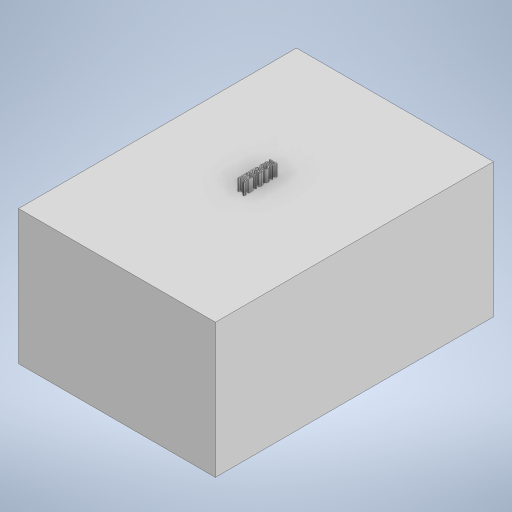
# Autodesk Inventor part: jetson
Saved by Autodesk Inventor 2023 (Build 270158000, 158)
## iProperties
Created: 2022-11-21
Part Number: jetson
Material: Genérico
Document SubType Name: Modeling
Designer: inigo
Density: 1 g/cm^3
Appearance: Valor por defecto
Author: inigo
Autodesk Inventor part; units mm, degrees
ref_plane "YZ Plane" through (0, 0, 0) normal (1, 0, 0) x (0, 1, 0)
ref_plane "XZ Plane" through (0, 0, 0) normal (0, 1, 0) x (-1, 0, 0)
ref_plane "XY Plane" through (0, 0, 0) normal (0, 0, 1) x (1, 0, 0)
sketch "Boceto1" plane through (0, 0, 0) normal (0, 1, 0) x (-1, 0, 0)
  line L0 (42.5, 60) -> (-42.5, 60)
  line L1 (-42.5, 60) -> (-42.5, -60)
  line L2 (-42.5, -60) -> (42.5, -60)
  line L3 (42.5, -60) -> (42.5, 60)
  line L4 (42.5, 60) -> (-42.5, -60) construction
  line L5 (-42.5, 60) -> (42.5, -60) construction
  point P0 (0, 0)
  dimension "d0" = 85
  dimension "d1" = 120
  constraints: 12 end point, 2 midpoint, 2 parallel, 1 horizontal, 1 perpendicular
  measures "d0" distance of L2.end L1.end
  measures "d1" distance of L1.end L0.end
extrude "Extrusión1" add sketch "Boceto1" along normal blind 58
sketch "Boceto2" plane through (0, 58, 0) normal (0, 1, 0) x (1, 0, 0)
  line L0 (-1.6968, -6.642) -> (-1.6968, 31.3478) construction
  line L1 (-1.6968, 31.3478) -> (74.717, 31.3478) construction
  line L2 (74.717, 31.3478) -> (74.717, -6.642) construction
  line L3 (74.717, -6.642) -> (-1.6968, -6.642) construction
  spline S0 degree 2 poles (0.6226, -5.1847) (1.0227, -5.1847) (1.4574, -5.6738) (1.4574, -6.0862) knots 0 0 0 1 2 2 2
  spline S1 degree 2 poles (1.4574, -6.0862) (1.4574, -6.185) (1.4229, -6.5136) (1.3982, -6.6247) knots 0 0 0 1 2 2 2
  line L4 (1.3982, -6.6247) -> (1.0079, -6.6247)
  line L5 (1.0079, -6.6247) -> (1.0079, -6.6025)
  spline S2 degree 2 poles (1.0079, -6.6025) (1.0375, -6.5185) (1.1067, -6.269) (1.1067, -6.1406) knots 0 0 0 1 2 2 2
  spline S3 degree 2 poles (1.1067, -6.1406) (1.1067, -5.9529) (1.0202, -5.7281) (0.9412, -5.6762) knots 0 0 0 1 2 2 2
  spline S4 degree 2 poles (0.9412, -5.6762) (0.8597, -5.6194) (0.6226, -5.5898) (0.467, -5.5898) knots 0 0 0 1 2 2 2
  line L6 (0.467, -5.5898) -> (-1.309, -5.5898)
  line L7 (-1.309, -5.5898) -> (-1.309, -6.2344)
  line L8 (-1.309, -6.2344) -> (-1.6326, -6.2344)
  line L9 (-1.6326, -6.2344) -> (-1.6326, -5.1847)
  line L10 (-1.6326, -5.1847) -> (0.6226, -5.1847)
  line L11 (1.4154, -4.5869) -> (-1.6326, -4.5869)
  line L12 (-1.6326, -4.5869) -> (-1.6326, -2.6801)
  line L13 (-1.6326, -2.6801) -> (-1.2719, -2.6801)
  line L14 (-1.2719, -2.6801) -> (-1.2719, -4.1819)
  line L15 (-1.2719, -4.1819) -> (-0.4371, -4.1819)
  line L16 (-0.4371, -4.1819) -> (-0.4371, -2.7814)
  line L17 (-0.4371, -2.7814) -> (-0.0764, -2.7814)
  line L18 (-0.0764, -2.7814) -> (-0.0764, -4.1819)
  line L19 (-0.0764, -4.1819) -> (1.0548, -4.1819)
  line L20 (1.0548, -4.1819) -> (1.0548, -2.6801)
  line L21 (1.0548, -2.6801) -> (1.4154, -2.6801)
  line L22 (1.4154, -2.6801) -> (1.4154, -4.5869)
  line L23 (1.4154, -1.5241) -> (-1.2719, -1.5241)
  line L24 (-1.2719, -1.5241) -> (-1.2719, -2.5467)
  line L25 (-1.2719, -2.5467) -> (-1.6326, -2.5467)
  line L26 (-1.6326, -2.5467) -> (-1.6326, -0.0965)
  line L27 (-1.6326, -0.0965) -> (-1.2719, -0.0965)
  line L28 (-1.2719, -0.0965) -> (-1.2719, -1.119)
  line L29 (-1.2719, -1.119) -> (1.4154, -1.119)
  line L30 (1.4154, -1.119) -> (1.4154, -1.5241)
  spline S5 degree 2 poles (1.4698, 1.062) (1.4698, 0.731) (1.3315, 0.2666) (1.2327, 0.0616) knots 0 0 0 1 2 2 2
  line L31 (1.2327, 0.0616) -> (0.7238, 0.0616)
  line L32 (0.7238, 0.0616) -> (0.7238, 0.0913)
  spline S6 degree 2 poles (0.7238, 0.0913) (0.9116, 0.2913) (1.119, 0.7977) (1.119, 1.0323) knots 0 0 0 1 2 2 2
  spline S7 degree 2 poles (1.119, 1.0323) (1.119, 1.3683) (0.8399, 1.7116) (0.6102, 1.7116) knots 0 0 0 1 2 2 2
  spline S8 degree 2 poles (0.6102, 1.7116) (0.4274, 1.7116) (0.2002, 1.5313) (0.1434, 1.3361) knots 0 0 0 1 2 2 2
  spline S9 degree 2 poles (0.1434, 1.3361) (0.1039, 1.1954) (0.0495, 0.9607) (0.0051, 0.7853) knots 0 0 0 1 2 2 2
  spline S10 degree 2 poles (0.0051, 0.7853) (-0.0369, 0.6273) (-0.1629, 0.3778) (-0.2642, 0.2815) knots 0 0 0 1 2 2 2
  spline S11 degree 2 poles (-0.2642, 0.2815) (-0.3654, 0.1876) (-0.6371, 0.0839) (-0.815, 0.0839) knots 0 0 0 1 2 2 2
  spline S12 degree 2 poles (-0.815, 0.0839) (-1.1855, 0.0839) (-1.6869, 0.6618) (-1.6869, 1.1089) knots 0 0 0 1 2 2 2
  spline S13 degree 2 poles (-1.6869, 1.1089) (-1.6869, 1.3658) (-1.5856, 1.8203) (-1.4893, 2.0154) knots 0 0 0 1 2 2 2
  line L33 (-1.4893, 2.0154) -> (-1.0052, 2.0154)
  line L34 (-1.0052, 2.0154) -> (-1.0052, 1.9858)
  spline S14 degree 2 poles (-1.0052, 1.9858) (-1.1386, 1.84) (-1.3362, 1.3856) (-1.3362, 1.1361) knots 0 0 0 1 2 2 2
  spline S15 degree 2 poles (-1.3362, 1.1361) (-1.3362, 0.8545) (-1.0719, 0.5062) (-0.857, 0.5062) knots 0 0 0 1 2 2 2
  spline S16 degree 2 poles (-0.857, 0.5062) (-0.6643, 0.5062) (-0.4346, 0.7112) (-0.3827, 0.9039) knots 0 0 0 1 2 2 2
  spline S17 degree 2 poles (-0.3827, 0.9039) (-0.3481, 1.0323) (-0.2592, 1.4053) (-0.2222, 1.5288) knots 0 0 0 1 2 2 2
  spline S18 degree 2 poles (-0.2222, 1.5288) (-0.1258, 1.8425) (0.2619, 2.134) (0.546, 2.134) knots 0 0 0 1 2 2 2
  spline S19 degree 2 poles (0.546, 2.134) (0.7263, 2.134) (1.0721, 1.9882) (1.1931, 1.8573) knots 0 0 0 1 2 2 2
  spline S20 degree 2 poles (1.1931, 1.8573) (1.3265, 1.7116) (1.4698, 1.3411) (1.4698, 1.062) knots 0 0 0 1 2 2 2
  spline S21 degree 2 poles (-1.2843, 4.7028) (-1.0817, 4.8757) (-0.4889, 5.0683) (-0.1086, 5.0683) knots 0 0 0 1 2 2 2
  spline S22 degree 2 poles (-0.1086, 5.0683) (0.2619, 5.0683) (0.8622, 4.8806) (1.0647, 4.7028) knots 0 0 0 1 2 2 2
  spline S23 degree 2 poles (1.0647, 4.7028) (1.2771, 4.5151) (1.4797, 4.0186) (1.4797, 3.7197) knots 0 0 0 1 2 2 2
  spline S24 degree 2 poles (1.4797, 3.7197) (1.4797, 3.411) (1.2697, 2.917) (1.0647, 2.7366) knots 0 0 0 1 2 2 2
  spline S25 degree 2 poles (1.0647, 2.7366) (0.8622, 2.5613) (0.2669, 2.3736) (-0.1086, 2.3736) knots 0 0 0 1 2 2 2
  spline S26 degree 2 poles (-0.1086, 2.3736) (-0.4914, 2.3736) (-1.0743, 2.5637) (-1.2843, 2.7391) knots 0 0 0 1 2 2 2
  spline S27 degree 2 poles (-1.2843, 2.7391) (-1.4868, 2.917) (-1.6968, 3.4134) (-1.6968, 3.7197) knots 0 0 0 1 2 2 2
  spline S28 degree 2 poles (-1.6968, 3.7197) (-1.6968, 4.0309) (-1.4794, 4.5299) (-1.2843, 4.7028) knots 0 0 0 1 2 2 2
  spline S29 degree 2 poles (-0.1086, 4.646) (-0.4099, 4.646) (-0.8767, 4.5151) (-1.0299, 4.3965) knots 0 0 0 1 2 2 2
  spline S30 degree 2 poles (-1.0299, 4.3965) (-1.188, 4.2755) (-1.346, 3.9346) (-1.346, 3.7222) knots 0 0 0 1 2 2 2
  spline S31 degree 2 poles (-1.346, 3.7222) (-1.346, 3.5024) (-1.1929, 3.1714) (-1.0299, 3.0454) knots 0 0 0 1 2 2 2
  spline S32 degree 2 poles (-1.0299, 3.0454) (-0.8743, 2.9244) (-0.405, 2.7959) (-0.1086, 2.7959) knots 0 0 0 1 2 2 2
  spline S33 degree 2 poles (-0.1086, 2.7959) (0.4917, 2.7959) (1.1289, 3.2998) (1.1289, 3.7222) knots 0 0 0 1 2 2 2
  spline S34 degree 2 poles (1.1289, 3.7222) (1.1289, 4.1446) (0.4917, 4.646) (-0.1086, 4.646) knots 0 0 0 1 2 2 2
  line L35 (1.4154, 7.694) -> (1.4154, 7.2395)
  line L36 (1.4154, 7.2395) -> (-1.2127, 5.8909)
  line L37 (-1.2127, 5.8909) -> (1.4154, 5.8909)
  line L38 (1.4154, 5.8909) -> (1.4154, 5.5129)
  line L39 (1.4154, 5.5129) -> (-1.6326, 5.5129)
  line L40 (-1.6326, 5.5129) -> (-1.6326, 6.0885)
  line L41 (-1.6326, 6.0885) -> (0.7807, 7.3161)
  line L42 (0.7807, 7.3161) -> (-1.6326, 7.3161)
  line L43 (-1.6326, 7.3161) -> (-1.6326, 7.694)
  line L44 (-1.6326, 7.694) -> (1.4154, 7.694)
  point P0 (0, 0)
  constraints: 2 other
extrude "Extrusión2" add sketch "Boceto2" along normal blind 5
